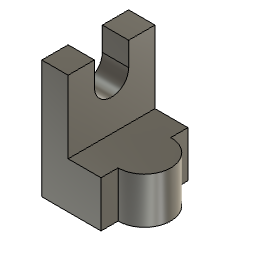
A1_AI22BTECH11005_1 (Autodesk Fusion 360 design; units mm, degrees)
Autodesk Fusion 360 part; units mm, degrees
sketch "Sketch1" plane through (0, 0, 0) normal (1, 0, 0) x (0, 1, 0)
  line L0 (0, 0) -> (66, 0)
  line L1 (66, 0) -> (66, 90)
  line L2 (66, 90) -> (46, 90)
  line L3 (20, 90) -> (0, 90)
  line L4 (0, 90) -> (0, 0)
  line L5 (20, 90) -> (20, 72)
  line L6 (46, 90) -> (46, 72)
  arc A0 (20, 72) -> (46, 72) centre (33, 72) ccw
  dimension "d1" = 66
  dimension "d2" = 90
  dimension "d3" = 20
  dimension "d5" = 20
  dimension "d6" = 18
  dimension "d7" = 18
  dimension "d8" = 13
  dimension "d9" = 90
  constraint horizontal L0
  constraint coincident L0.start L4.end
  constraint perpendicular L0 L1
  constraint horizontal L2
  constraint perpendicular L0 L4
  constraint vertical L6
  constraint tangent L5 A0
  measures "d1" distance of L0.start L0.end
  measures "d2" distance of L0.end L1.end
  measures "d3" distance of L1.end L2.end
  measures "d5" distance of L3.start L3.end
  measures "d6" distance of L3.start L5.end
  measures "d7" distance of L2.end L6.end
  measures "d8" radius of A0
  measures "d9" distance of L3.end L0.start
extrude "Extrude1" add sketch "Sketch1" along normal blind 20
sketch "Sketch2" plane through (0, 0, 0) normal (0, 0, 1) x (1, 0, 0)
  line L0 (0, 0) -> (45, 0)
  line L1 (0, 0) -> (0, 66)
  line L2 (0, 66) -> (45, 66)
  line L3 (45, 66) -> (45, 53)
  line L4 (45, 13) -> (45, 0)
  arc A0 (45, 13) -> (45, 53) centre (45, 33) ccw
  dimension "d13" = 66
  dimension "d14" = 45
  dimension "d15" = 13
  dimension "d18" = 13
  dimension "d20" = 40
  constraint horizontal L0
  constraint coincident L0.start L1.start
  constraint perpendicular L0 L1
  constraint perpendicular L1 L2
  constraint vertical L3
  constraint vertical L4
  measures "d13" distance of L0.start L1.end
  measures "d14" distance of L1.end L2.end
  measures "d15" distance of L2.end L3.end
  measures "d18" distance of L0.end L4.start
  measures "d20" diameter of A0
extrude "Extrude2" add sketch "Sketch2" along normal blind 35
